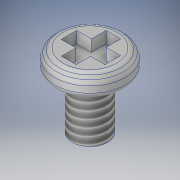
# Autodesk Inventor part: sqrew base
Saved by Autodesk Inventor 2018 (Build 220112000, 112)
## iProperties
Created: 2018-03-02
Part Number: sqrew base
Material: Aluminum 6061
Document SubType Name: Modeling
Designer: 238438
Density: 2.7 g/cm^3
Appearance: Aluminum - Flat
Mass: 0.386382 g
Surface Area: 2.19739 cm^2
Volume: 0.143104 cm^3
Author: 238438
Autodesk Inventor part; units mm, degrees
ref_plane "YZ Plane" through (0, 0, 0) normal (1, 0, 0) x (0, 1, 0)
ref_plane "XZ Plane" through (0, 0, 0) normal (0, 1, 0) x (-1, 0, 0)
ref_plane "XY Plane" through (0, 0, 0) normal (0, 0, 1) x (1, 0, 0)
sketch "Sketch1" plane through (0, 0, 0) normal (0, 0, 1) x (1, 0, 0)
  line L0 (0, 0) -> (3.81, 0)
  line L1 (3.81, 0) -> (3.81, -2.2225)
  line L2 (3.81, -2.2225) -> (1.905, -2.2225)
  line L3 (1.905, -2.2225) -> (1.905, -7.9375)
  line L4 (1.905, -7.9375) -> (0, -7.9375)
  line L5 (0, -7.9375) -> (0, 0)
  line L6 (0, 0) -> (0, -14.1407)
  dimension "d0" = 3.81
  dimension "d1" = 2.2225
  dimension "d2" = 1.905
  dimension "d3" = 5.715
  dimension "d4" = 90
  constraints: 14 end point, 4 perpendicular, 2 horizontal, 1 point on line
  measures "d0" distance of L0.start L0.end
  measures "d1" distance of L0.end L1.end
  measures "d2" distance of L1.end L2.end
  measures "d3" distance of L2.end L3.end
  measures "d4" angle of L3 L2
revolve "Revolution1" add sketch "Sketch1" angle 360 about axis through (0, 0, 0) along (0, -1, 0)
chamfer "Chamfer1" distance 0.635 angle 45 1 edges at (-3.81, 0, 0)
fillet "Fillet1" radius 0.635 3 edges at (-3.175, 0, 0) (-3.81, -0.635, 0) (-3.81, -2.2225, 0)
thread "Thread1" size "8-32 UNC" class "2A" standard "ANSI Unified Screw Threads" full length
sketch "Sketch2" plane through (0, 0, 0) normal (0, 1, 0) x (1, 0, 0)
  line L0 (-0.752, -2.3428) -> (0.8388, -2.3428)
  line L1 (0.8388, 2.4875) -> (-0.752, 2.4875)
  line L2 (2.4007, -0.7809) -> (2.4007, 0.8966)
  line L3 (-2.3428, 0.8966) -> (-2.3428, -0.7809)
  line L4 (-2.3428, -0.7809) -> (-0.752, -0.7809)
  line L5 (0.8388, -0.7809) -> (2.4007, -0.7809)
  line L6 (2.4007, 0.8966) -> (0.8388, 0.8966)
  line L7 (-0.752, 0.8966) -> (-2.3428, 0.8966)
  line L8 (-0.752, 2.4875) -> (-0.752, 0.8966)
  line L9 (-0.752, -0.7809) -> (-0.752, -2.3428)
  line L10 (0.8388, -2.3428) -> (0.8388, -0.7809)
  line L11 (0.8388, 0.8966) -> (0.8388, 2.4875)
  point P0 (0, 0)
  constraints: 24 end point, 10 parallel, 4 perpendicular, 3 horizontal
extrude "Extrusion1" cut sketch "Sketch2" against normal blind 1.27
body "Solid1"
